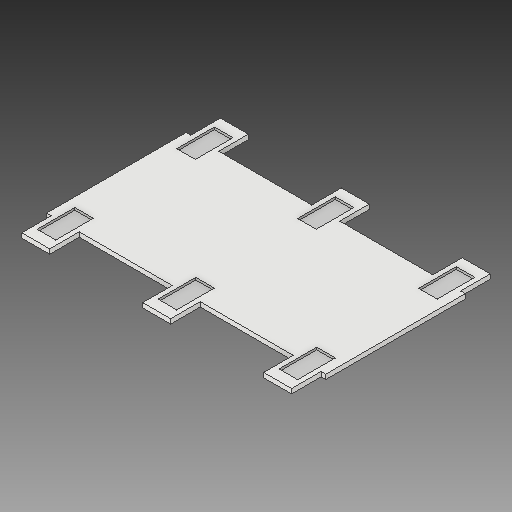
# Autodesk Inventor part: Body_Top
Saved by Autodesk Inventor 2017 (Build 210142000, 142)
## iProperties
Created: 2017-01-25
Part Number: Body_Top
Material: Generic
Document SubType Name: Modeling
Designer: Alexander Miller
Density: 1 g/cm^3
Appearance: Default
Author: Alexander Miller
Autodesk Inventor part; units mm, degrees
ref_plane "YZ Plane" through (0, 0, 0) normal (1, 0, 0) x (0, 1, 0)
ref_plane "XZ Plane" through (0, 0, 0) normal (0, 1, 0) x (-1, 0, 0)
ref_plane "XY Plane" through (0, 0, 0) normal (0, 0, 1) x (1, 0, 0)
sketch "Sketch1" plane through (0, 0, 0) normal (0, 1, 0) x (-1, 0, 0)
  line L0 (-150, 0) -> (-150, -75)
  line L1 (-150, -75) -> (-145, -75)
  line L2 (-145, -75) -> (-145, -106.75)
  line L3 (-145, -106.75) -> (-115, -106.75)
  line L4 (-115, -106.75) -> (-115, -75)
  line L5 (-115, -75) -> (-15, -75)
  line L6 (-15, -75) -> (-15, -106.75)
  line L7 (-15, -106.75) -> (15, -106.75)
  line L8 (15, -106.75) -> (15, -75)
  line L9 (15, -75) -> (115, -75)
  line L10 (115, -75) -> (115, -106.75)
  line L11 (115, -106.75) -> (145, -106.75)
  line L12 (145, -106.75) -> (145, -75)
  line L13 (145, -75) -> (150, -75)
  line L14 (150, -75) -> (150, 0)
  line L15 (112, 0) -> (-112, 0) projected
  line L16 (-150, 0) -> (-150, 75)
  line L17 (-150, 75) -> (-145, 75)
  line L18 (-145, 75) -> (-145, 106.75)
  line L19 (-145, 106.75) -> (-115, 106.75)
  line L20 (-115, 106.75) -> (-115, 75)
  line L21 (-115, 75) -> (-15, 75)
  line L22 (-15, 75) -> (-15, 106.75)
  line L23 (-15, 106.75) -> (15, 106.75)
  line L24 (15, 106.75) -> (15, 75)
  line L25 (15, 75) -> (115, 75)
  line L26 (115, 75) -> (115, 106.75)
  line L27 (115, 106.75) -> (145, 106.75)
  line L28 (145, 106.75) -> (145, 75)
  line L29 (145, 75) -> (150, 75)
  line L30 (150, 75) -> (150, 0)
  point P0 (0, 0)
  point P1 (0, -106.75)
  dimension "d0" = 30
  dimension "d1" = 75
  dimension "d2" = 31.75
  dimension "d3" = 5
  dimension "d4" = 100
  constraints: 60 end point, 18 point on line, 14 symmetric about line, 9 perpendicular, 5 equal length, 2 vertical, 1 horizontal alignment, 1 midpoint, 1 vertical alignment
  measures "d0" distance of L10.end L11.end
  measures "d1" distance of L13.end L14.end
  measures "d2" distance of L11.end L12.end
  measures "d3" distance of L12.end L13.end
  measures "d4" distance of L8.end L9.end
extrude "Extrusion1" add sketch "Sketch1" along normal blind 5
sketch "Sketch2" plane through (0, 5, 0) normal (0, 1, 0) x (1, 0, 0)
  line L0 (-120, 54.75) -> (-140, 54.75)
  line L1 (-140, 54.75) -> (-140, 95.25)
  line L2 (-140, 95.25) -> (-120, 95.25)
  line L3 (-120, 95.25) -> (-120, 54.75)
  line L4 (10, 54.75) -> (-10, 54.75)
  line L5 (-10, 54.75) -> (-10, 95.25)
  line L6 (-10, 95.25) -> (10, 95.25)
  line L7 (10, 95.25) -> (10, 54.75)
  line L8 (140, 54.75) -> (120, 54.75)
  line L9 (120, 54.75) -> (120, 95.25)
  line L10 (120, 95.25) -> (140, 95.25)
  line L11 (140, 95.25) -> (140, 54.75)
  line L12 (-210, 0) -> (210, 0) projected
  line L13 (-120, -54.75) -> (-140, -54.75)
  line L14 (-140, -54.75) -> (-140, -95.25)
  line L15 (-140, -95.25) -> (-120, -95.25)
  line L16 (-120, -95.25) -> (-120, -54.75)
  line L17 (10, -54.75) -> (-10, -54.75)
  line L18 (-10, -54.75) -> (-10, -95.25)
  line L19 (-10, -95.25) -> (10, -95.25)
  line L20 (10, -95.25) -> (10, -54.75)
  line L21 (140, -54.75) -> (120, -54.75)
  line L22 (120, -54.75) -> (120, -95.25)
  line L23 (120, -95.25) -> (140, -95.25)
  line L24 (140, -95.25) -> (140, -54.75)
  line L25 (-115, 106.75) -> (-145, 106.75) projected
  line L26 (-145, 106.75) -> (-145, 75) projected
  line L27 (-15, 106.75) -> (-15, 75) projected
  line L28 (115, 106.75) -> (115, 75) projected
  point P0 (0, 0)
  dimension "d7" = 11.5
  dimension "d8" = 5
  dimension "d9" = 20
  dimension "d10" = 40.5
  dimension "d11" = 5
  dimension "d12" = 5
  constraints: 48 end point, 12 symmetric about line, 6 parallel, 4 point on line, 3 horizontal, 3 perpendicular, 2 collinear, 2 horizontal alignment
  measures "d7" distance between parallel lines of L2 L25
  measures "d8" distance between parallel lines of L1 L26
  measures "d9" distance of L1.end L2.end
  measures "d10" distance of L2.end L0.start
  measures "d11" distance between parallel lines of L27 L5
  measures "d12" distance between parallel lines of L9 L28
extrude "Extrusion2" cut sketch "Sketch2" against normal blind 2.5
equation "\"d0\" = servo_depth + 2 * material_thickness"
equation "\"d1\" = 0.5 * body_width"
equation "\"d2\" = servo_mount_length + 0.5 * servo_width + material_thickness"
equation "\"d4\" = leg_distance"
equation "\"d5\" = material_thickness"
equation "\"d7\" = material_thickness + servo_mount_length"
equation "\"d8\" = material_thickness"
equation "\"d9\" = servo_depth"
equation "\"d10\" = servo_width"
equation "\"d11\" = d8"
equation "\"d12\" = d8"
equation "\"d13\" = 0.5 * material_thickness"
equation "\"material_thickness\" = material_thickness_1"
equation "\"leg_distance\" = leg_distance_1"
equation "\"servo_depth\" = 20"
equation "\"body_width\" = 150"
equation "\"servo_mount_length\" = 6.5"
equation "\"servo_width\" = 40.5"
equation "\"material_thickness_1\" = 5"
equation "\"leg_distance_1\" = 100"
body "Solid1"
